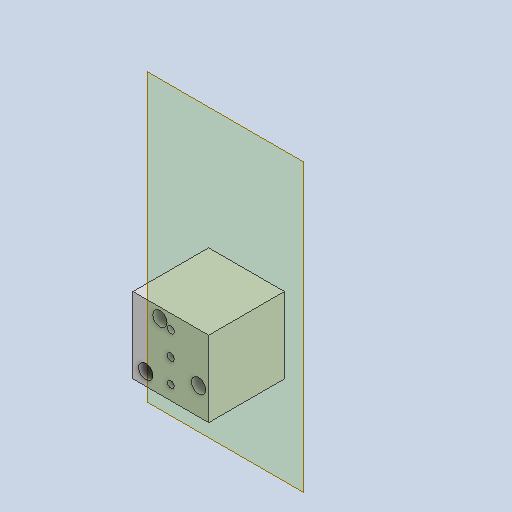
# Autodesk Inventor part: 30_XY_Sample_lightsheetarm_sample_screwadapter_v3
Saved by Autodesk Inventor 2022 (Build 260153000, 153)
## iProperties
Created: 2021-12-01
Part Number: 30_XY_Sample_lightsheetarm_sample_screwadapter_v3
Material: Generisch
Document SubType Name: Modeling
Designer: diederichbenedict
Density: 1 g/cm^3
Appearance: Vorgabe
Author: diederichbenedict
Autodesk Inventor part; units mm, degrees
ref_plane "YZ Plane" through (0, 0, 0) normal (1, 0, 0) x (0, 1, 0)
ref_plane "XZ Plane" through (0, 0, 0) normal (0, 1, 0) x (-1, 0, 0)
ref_plane "XY Plane" through (0, 0, 0) normal (0, 0, 1) x (1, 0, 0)
ref_plane "Arbeitsebene1" through (0, 0, -8) normal (0, 0, -1) x (-1, 0, 0)
sketch "Skizze1" plane through (0, 0, -8) normal (0, 0, -1) x (-1, 0, 0)
  line L0 (-30, -73.2876) -> (-18.6416, -61.9292) projected
  line L1 (-18.6416, -61.9292) -> (-17.5809, -62.9898) projected
  line L2 (-17.5809, -62.9898) -> (-30, -75.4089) projected
  line L3 (-30, -75.4089) -> (-30, -76) projected
  arc A0 (-30, -76) -> (-26, -80) centre (-26, -76) ccw projected
  line L4 (-18, -80) -> (-26, -80) projected
  arc A1 (-18, -80) -> (-14, -76) centre (-18, -76) ccw projected
  line L5 (-14, -34) -> (-14, -76) projected
  arc A2 (-10, -30) -> (-14, -34) centre (-10, -34) ccw projected
  line L6 (-10, -30) -> (12, -30) projected
  arc A3 (16, -34) -> (12, -30) centre (12, -34) ccw projected
  line L7 (16, -34) -> (16, -76) projected
  arc A4 (16, -76) -> (20, -80) centre (20, -76) ccw projected
  line L8 (20, -80) -> (26, -80) projected
  arc A5 (26, -80) -> (30, -76) centre (26, -76) ccw projected
  line L9 (30, 28) -> (30, -76) projected
  line L10 (30, 28) -> (28, 30) projected
  line L11 (28, 30) -> (-28, 30) projected
  line L12 (-28, 30) -> (-30, 28) projected
  line L13 (-30, 28) -> (-30, -73.2876) projected
  circle A6 centre (-10, -25) radius 1.45 projected
  circle A7 centre (-10, 25) radius 1.45 projected
  circle A8 centre (10, 25) radius 1.45 projected
  circle A9 centre (10, -25) radius 1.45 projected
  circle A10 centre (25, -10) radius 1.45 projected
  circle A11 centre (-25, -10) radius 1.45 projected
  circle A12 centre (-25, 10) radius 1.45 projected
  circle A13 centre (25, 10) radius 1.45 projected
  circle A14 centre (-17.5, -17.5) radius 1.95 projected
  circle A15 centre (17.5, 17.5) radius 1.95 projected
  circle A16 centre (17.5, -17.5) radius 1.95 projected
  circle A17 centre (-17.5, 17.5) radius 1.95 projected
  circle A18 centre (-25, 25) radius 2.325 projected
  circle A19 centre (25, -25) radius 2.325 projected
  circle A20 centre (-25, -25) radius 2.325 projected
  circle A21 centre (25, 25) radius 2.325 projected
  circle A22 centre (0, 0) radius 16 projected
  circle A23 centre (23, -74) radius 3.75 projected
  circle A24 centre (23, -64) radius 1.45 projected
  circle A25 centre (23, -54) radius 1.45 projected
  line L14 (7, -80) -> (39, -80)
  line L15 (39, -80) -> (39, -48)
  line L16 (39, -48) -> (7, -48)
  line L17 (7, -48) -> (7, -80)
  line L18 (7, -80) -> (39, -48) construction
  line L19 (39, -80) -> (7, -48) construction
  circle A26 centre (23, -74) radius 1.4
  line L20 (34.516, -58.7768) -> (32.4244, -50.9708) projected
  line L21 (24.0592, -48.7293) -> (7.7293, -65.0592) projected
  line L22 (9.9708, -73.4244) -> (17.7768, -75.516) projected
  circle A27 centre (24.1439, -65.1439) radius 11.6667
  arc A28 (7.7293, -65.0592) -> (9.9708, -73.4244) centre (11.2649, -68.5948) ccw projected
  line L23 (34.516, -58.7768) -> (17.7768, -75.516) projected
  arc A29 (32.4244, -50.9708) -> (24.0592, -48.7293) centre (27.5948, -52.2649) ccw projected
  point P0 (0, 0)
  point P1 (26, -80)
  point P2 (16, -48)
  point P3 (16, -56.7886)
  point P4 (19.8793, -76.0794)
  point P5 (24.6629, -77.3611)
  point P6 (24.985, -48)
  point P7 (7, -65.985)
  point P8 (7, -71.2045)
  point P9 (30.2045, -48)
  dimension "d0" = 32
  dimension "d1" = 32
  dimension "d2" = 2.8
  constraints: 12 end point, 3 tangent, 2 centre point, 2 midpoint, 2 parallel, 1 coincident, 1 horizontal, 1 perpendicular
  measures "d0" distance of L16.end L15.end
  measures "d1" distance of L15.end L14.end
  measures "d2" diameter of A26
extrude "Extrusion1" add sketch "Skizze1" along normal blind 32 contours L16 A29 L20 L23 A27 L9 | L9 A27 A25 L21 A29 L16 | L16 L15 L14 A5 L9 A27 L23 L20 A29 | A29 L21 L7 L16 | A27 L23 L9 | L9 L23 A23 A27 L7 A25 | L7 L21 A28 L17 L16 | L23 A27 L9 | L9 A27 A23 L23 | A27 L7 L22 A28 L17 L21 | L7 A27 | L9 A5 L8 A4 L7 L22 L23 A27 A23 | L23 A23 | A23 A27 L23 | A27 L23 L22 L7 | A23 A27 | A23 A27 L23 | L14 L17 A28 L22 L7 A4
sketch "Skizze2" plane through (0, 0, -8) normal (0, 0, -1) x (-1, 0, 0)
  circle A0 centre (33.5719, -74.5719) radius 1.4
  line L0 (33.5719, -74.5719) -> (11.2649, -68.5948)
  line L1 (11.2649, -68.5948) -> (27.5948, -52.2649)
  line L2 (27.5948, -52.2649) -> (33.5719, -74.5719)
  line L3 (9.7029, -90.6426) -> (49.4807, -50.8648) construction
  line L4 (-4.7029, -89.492) -> (48.3301, -36.459) construction
  line L5 (39, -80) -> (39, -48) construction
  line L6 (7, -48) -> (7, -80) construction
  line L7 (39, -80) -> (7, -48) construction
  arc A1 (32.4244, -50.9708) -> (24.0592, -48.7293) centre (27.5948, -52.2649) ccw projected
  line L8 (24.0592, -48.7293) -> (7.7293, -65.0592) projected
  arc A2 (7.7293, -65.0592) -> (9.9708, -73.4244) centre (11.2649, -68.5948) ccw projected
  line L9 (9.9708, -73.4244) -> (32.2778, -79.4016) projected
  arc A3 (32.2778, -79.4016) -> (38.4016, -73.2778) centre (33.5719, -74.5719) ccw projected
  line L10 (38.4016, -73.2778) -> (32.4244, -50.9708) projected
  point P0 (0, 0)
  point P1 (24.4298, -55.4298)
  point P2 (24.1439, -65.1439)
  constraints: 8 end point, 2 point on line, 1 centre point, 1 parallel, 5 other
hole "Bohrung1" at (-27.5948, -52.2649, -8) at (-11.2649, -68.5948, -8) at (-33.5719, -74.5719, -8) direction (0, 0, -1) diameter 2.8 end through all counterbore diameter 6 counterbore depth 25
sketch "Skizze4" plane through (-32.4244, -50.9708, -40) normal (-0.9659, 0.2588, 0) x (0, 0, 1)
  line L0 (6.9, -13.047) -> (-22.6933, -13.047)
  line L1 (6.9, -10.047) -> (-22.6933, -10.047)
  circle A0 centre (4.5207, -11.5212) radius 1.4
  point P0 (40, 57.626)
  dimension "d19" = 2.8
  constraints: 4 end point, 2 horizontal, 1 centre point, 4 other
  measures "d19" diameter of A0
extrude "Extrusion3" [suppressed]
sketch "Skizze5" plane through (0, 0, -40) normal (0, 0, -1) x (-1, 0, 0)
  line L0 (9.9708, -73.4244) -> (17.7768, -75.516) projected
  line L1 (24.0592, -48.7293) -> (7.7293, -65.0592) projected
  line L2 (34.516, -58.7768) -> (32.4244, -50.9708) projected
  circle A0 centre (24.1439, -65.1439) radius 11.6667
  circle A1 centre (24.1439, -65.1439) radius 0.5
  point P0 (0, 0)
  dimension "d22" = 1
  constraints: 3 tangent, 2 centre point, 1 coincident
  measures "d22" diameter of A1
extrude "Extrusion4" cut sketch "Skizze5" against normal blind 1 contours A1
pattern_circular "Runde Anordnung2" [suppressed]
